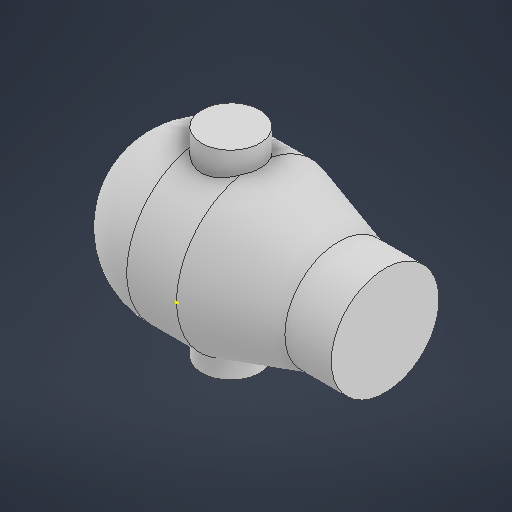
# Autodesk Inventor part: diff
Saved by Autodesk Inventor 2026.2 (Build 302298010, 298A)
## iProperties
Created: 2026-07-07
Part Number: diff
Material: Generic
Document SubType Name: Modeling
Designer: tasle
Density: 1.48334 g/cm^3
Appearance: Default
Mass: 23000 g
Surface Area: 3285.73 cm^2
Volume: 15505.6 cm^3
Author: tasle
Autodesk Inventor part; units mm, degrees
ref_plane "YZ Plane" through (0, 0, 0) normal (1, 0, 0) x (0, 1, 0)
ref_plane "XZ Plane" through (0, 0, 0) normal (0, 1, 0) x (-1, 0, 0)
ref_plane "XY Plane" through (0, 0, 0) normal (0, 0, 1) x (1, 0, 0)
sketch "Sketch1" plane through (0, 0, 0) normal (0, 1, 0) x (-1, 0, 0)
  line L0 (0, 0) -> (60, 0)
  line L1 (60, 0) -> (60, -190.5)
  line L2 (60, -190.5) -> (0, -190.5)
  line L3 (0, -190.5) -> (0, 0)
  line L4 (-100, -30.4611) -> (-155.9, -30.4611)
  line L5 (-155.9, -30.4611) -> (-155.9, -160.3726)
  line L6 (-155.9, -160.3726) -> (-100, -160.3726)
  line L7 (-100, -160.3726) -> (-100, -30.4611)
  line L8 (0, -95.25) -> (-100, -95.25)
  line L9 (-100, -160.3726) -> (0, -190.5)
  arc A0 (60, -190.5) -> (60, 0) centre (60, -95.25) ccw
  line L10 (0, 0) -> (-100, -30.4611)
  line L11 (-155.9, -95.4169) -> (155.25, -95.25)
  point P0 (-100, -95.3869)
  point P1 (0, -95.3333)
  dimension "d0" = 190.5
  dimension "d1" = 60
  dimension "d2" = 100
  dimension "d8" = 311.15
  dimension "d9" = 129.9115
  constraints: 24 end point, 4 parallel, 3 horizontal, 3 midpoint, 3 point on circle, 2 perpendicular, 1 centre point, 1 point on line
  measures "d0" distance of L0.end L1.end
  measures "d1" distance of L1.end L2.end
  measures "d2" distance of L8.start L8.end
  measures "d8" distance of L11.start L11.end
  measures "d9" distance of L4.end L5.end
revolve "Revolution1" add sketch "Sketch1" angle 360 about axis through (155.9, 0, -95.4169) along (-0.9999999, 0, 0.0005362) picked at (64.5185, -32.0902) contours L0 L1 L11 L3 | L3 L8 L7 L10 | A0 L11 L1 | L7 L11 L5 L4
sketch "Sketch2" plane through (0, 0, 0) normal (0, 1, 0) x (-1, 0, 0)
  point P0 (0, 0)
sketch "Sketch3" plane through (0, 0, 0) normal (0, 1, 0) x (-1, 0, 0)
  circle A0 centre (30.0512, -95.3843) radius 35
  line L0 (0.1022, -190.6665) -> (0, 0) projected
  line L1 (30.0512, -95.3843) -> (30.1022, -190.6343)
  line L2 (0.1022, -190.6665) -> (60.1022, -190.6021) projected
  dimension "d4" = 70
  dimension "d5" = 30
  dimension "d10" = 95.25
  constraints: 2 end point, 1 centre point, 1 midpoint
  measures "d4" diameter of A0
  measures "d5" distance from line of L0 L1.start
  measures "d10" distance of L1.start L1.end
extrude "Extrusion1" add sketch "Sketch3" along normal mid plane 239.7 contours A0 L0 | L0 A0
body "Solid1"
